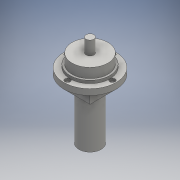
# Autodesk Inventor part: TukasaMoter
Saved by Autodesk Inventor 2016 (Build 200138000, 138)
## iProperties
Created: 2016-11-23
Part Number: TukasaMoter
Material: 一般
Document SubType Name: Modeling
Designer: Daisuke
Density: 1 g/cm^3
Appearance: 既定
Author: Daisuke
Autodesk Inventor part; units mm, degrees
ref_plane "YZ Plane" through (0, 0, 0) normal (1, 0, 0) x (0, 1, 0)
ref_plane "XZ Plane" through (0, 0, 0) normal (0, 1, 0) x (-1, 0, 0)
ref_plane "XY Plane" through (0, 0, 0) normal (0, 0, 1) x (1, 0, 0)
sketch "スケッチ1" plane through (0, 0, 0) normal (0, 0, 1) x (1, 0, 0)
  circle A0 centre (0, 0) radius 17
  dimension "d0" = 34
  constraints: 1 centre point, 1 coincident
  measures "d0" diameter of A0
extrude "押し出し1" add sketch "スケッチ1" along normal blind 73
sketch "スケッチ2" plane through (0, 0, 73) normal (0, 0, 1) x (1, 0, 0)
  line L0 (-21.5, 21.5) -> (21.5, 21.5)
  line L1 (21.5, 21.5) -> (21.5, -21.5)
  line L2 (21.5, -21.5) -> (-21.5, -21.5)
  line L3 (-21.5, -21.5) -> (-21.5, 21.5)
  line L4 (-21.5, 21.5) -> (21.5, -21.5) construction
  line L5 (21.5, 21.5) -> (-21.5, -21.5) construction
  point P0 (0, 0)
  dimension "d3" = 43
  dimension "d4" = 43
  constraints: 12 end point, 2 midpoint, 2 parallel, 1 horizontal, 1 perpendicular
  measures "d3" distance of L1.end L2.end
  measures "d4" distance of L0.end L1.end
extrude "押し出し2" add sketch "スケッチ2" along normal blind 18.5
sketch "スケッチ3" plane through (0, 0, 91.5) normal (0, 0, 1) x (1, 0, 0)
  circle A0 centre (0, 0) radius 40
  dimension "d7" = 80
  constraints: 1 centre point, 1 coincident
  measures "d7" diameter of A0
extrude "押し出し3" add sketch "スケッチ3" along normal blind 9
sketch "スケッチ4" plane through (0, 0, 100.5) normal (0, 0, 1) x (1, 0, 0)
  circle A0 centre (0, 0) radius 30.5
  dimension "d10" = 61
  constraints: 1 centre point, 1 coincident
  measures "d10" diameter of A0
extrude "押し出し4" add sketch "スケッチ4" along normal blind 4.5
sketch "スケッチ5" plane through (0, 0, 105) normal (0, 0, 1) x (1, 0, 0)
  circle A0 centre (0, 0) radius 27.5
  dimension "d13" = 55
  constraints: 1 centre point, 1 coincident
  measures "d13" diameter of A0
extrude "押し出し5" add sketch "スケッチ5" along normal blind 15
sketch "スケッチ6" plane through (0, 0, 120) normal (0, 0, 1) x (1, 0, 0)
  circle A0 centre (0, 0) radius 6
  dimension "d16" = 12
  constraints: 1 centre point, 1 coincident
  measures "d16" diameter of A0
extrude "押し出し6" add sketch "スケッチ6" along normal blind 21
sketch "スケッチ7" plane through (0, 0, 100.5) normal (0, 0, 1) x (1, 0, 0)
  circle A0 centre (0, 0) radius 34.5 construction
  circle A1 centre (-34.5, 0) radius 2
  circle A2 centre (0, -34.5) radius 2
  circle A3 centre (34.5, 0) radius 2
  circle A4 centre (0, 34.5) radius 2
  dimension "d19" = 69
  dimension "d20" = 4
  dimension "d23" = 360
  constraints: 4 centre point, 1 coincident, 1 horizontal alignment, 11 other
  measures "d20" diameter of A1
extrude "押し出し7" cut sketch "スケッチ7" against normal blind 9
sketch "スケッチ8" plane through (0, 0, 100.5) normal (0, 0, 1) x (1, 0, 0)
  circle A0 centre (0, 0) radius 34.5 construction
  circle A1 centre (-34.5, 0) radius 4
  circle A2 centre (0, -34.5) radius 4
  circle A3 centre (34.5, 0) radius 4
  circle A4 centre (0, 34.5) radius 4
  dimension "d27" = 69
  dimension "d28" = 8
  dimension "d31" = 360
  constraints: 4 centre point, 1 coincident, 1 horizontal alignment, 11 other
  measures "d28" diameter of A1
extrude "押し出し8" cut sketch "スケッチ8" against normal blind 4
